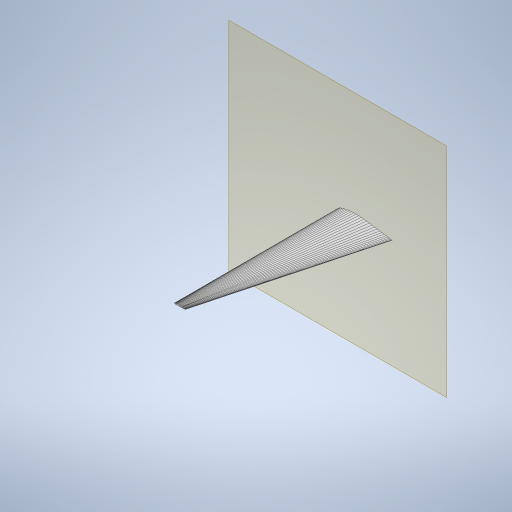
# Autodesk Inventor part: Część3
Saved by Autodesk Inventor 2023 (Build 270158000, 158)
## iProperties
Created: 2024-01-30
Part Number: Część3
Material: Ogólny
Document SubType Name: Modeling
Designer: domin
Density: 1 g/cm^3
Appearance: Domyślna
Author: domin
Autodesk Inventor part; units mm, degrees
ref_plane "YZ Plane" through (0, 0, 0) normal (1, 0, 0) x (0, 1, 0)
ref_plane "XZ Plane" through (0, 0, 0) normal (0, 1, 0) x (-1, 0, 0)
sketch "Szkic1" plane through (0, 0, 0) normal (0, 0, 1) x (1, 0, 0)
  line L0 (1, 0) -> (0.9965, 0.0005)
  line L1 (0.9965, 0.0005) -> (0.9863, 0.002)
  line L2 (0.9863, 0.002) -> (0.9701, 0.0049)
  line L3 (0.9701, 0.0049) -> (0.9487, 0.0088)
  line L4 (0.9487, 0.0088) -> (0.9224, 0.0134)
  line L5 (0.9224, 0.0134) -> (0.8913, 0.0184)
  line L6 (0.8913, 0.0184) -> (0.8558, 0.024)
  line L7 (0.8558, 0.024) -> (0.8163, 0.0301)
  line L8 (0.8163, 0.0301) -> (0.7736, 0.0367)
  line L9 (0.7736, 0.0367) -> (0.7281, 0.0435)
  line L10 (0.7281, 0.0435) -> (0.6804, 0.0506)
  line L11 (0.6804, 0.0506) -> (0.6313, 0.0576)
  line L12 (0.6313, 0.0576) -> (0.5814, 0.0644)
  line L13 (0.5814, 0.0644) -> (0.5313, 0.0708)
  line L14 (0.5313, 0.0708) -> (0.4817, 0.0764)
  line L15 (0.4817, 0.0764) -> (0.4331, 0.0808)
  line L16 (0.4331, 0.0808) -> (0.3857, 0.0836)
  line L17 (0.3857, 0.0836) -> (0.3398, 0.0848)
  line L18 (0.3398, 0.0848) -> (0.2957, 0.0843)
  line L19 (0.2957, 0.0843) -> (0.2536, 0.0821)
  line L20 (0.2536, 0.0821) -> (0.2137, 0.0782)
  line L21 (0.2137, 0.0782) -> (0.1762, 0.073)
  line L22 (0.1762, 0.073) -> (0.1416, 0.0667)
  line L23 (0.1416, 0.0667) -> (0.1102, 0.0594)
  line L24 (0.1102, 0.0594) -> (0.0823, 0.0514)
  line L25 (0.0823, 0.0514) -> (0.0581, 0.0428)
  line L26 (0.0581, 0.0428) -> (0.0379, 0.0338)
  line L27 (0.0379, 0.0338) -> (0.0219, 0.0247)
  line L28 (0.0219, 0.0247) -> (0.0102, 0.0157)
  line L29 (0.0102, 0.0157) -> (0.0028, 0.0071)
  line L30 (0.0028, 0.0071) -> (0, -0.0001)
  line L31 (0, -0.0001) -> (0.003, -0.0063)
  line L32 (0.003, -0.0063) -> (0.0121, -0.012)
  line L33 (0.0121, -0.012) -> (0.0263, -0.0175)
  line L34 (0.0263, -0.0175) -> (0.0454, -0.0223)
  line L35 (0.0454, -0.0223) -> (0.0694, -0.0265)
  line L36 (0.0694, -0.0265) -> (0.0981, -0.0299)
  line L37 (0.0981, -0.0299) -> (0.1311, -0.0326)
  line L38 (0.1311, -0.0326) -> (0.1682, -0.0345)
  line L39 (0.1682, -0.0345) -> (0.2089, -0.0357)
  line L40 (0.2089, -0.0357) -> (0.2529, -0.0361)
  line L41 (0.2529, -0.0361) -> (0.2997, -0.0359)
  line L42 (0.2997, -0.0359) -> (0.3486, -0.0349)
  line L43 (0.3486, -0.0349) -> (0.3994, -0.033)
  line L44 (0.3994, -0.033) -> (0.4517, -0.0304)
  line L45 (0.4517, -0.0304) -> (0.505, -0.0274)
  line L46 (0.505, -0.0274) -> (0.5586, -0.0243)
  line L47 (0.5586, -0.0243) -> (0.6119, -0.021)
  line L48 (0.6119, -0.021) -> (0.6641, -0.0179)
  line L49 (0.6641, -0.0179) -> (0.7147, -0.0149)
  line L50 (0.7147, -0.0149) -> (0.7628, -0.0121)
  line L51 (0.7628, -0.0121) -> (0.808, -0.0096)
  line L52 (0.808, -0.0096) -> (0.8495, -0.0074)
  line L53 (0.8495, -0.0074) -> (0.8868, -0.0056)
  line L54 (0.8868, -0.0056) -> (0.9194, -0.0039)
  line L55 (0.9194, -0.0039) -> (0.947, -0.0024)
  line L56 (0.947, -0.0024) -> (0.9693, -0.0011)
  line L57 (0.9693, -0.0011) -> (0.986, -0.0003)
  line L58 (0.986, -0.0003) -> (0.9964, 0)
  line L59 (0.9964, 0) -> (1, 0)
  point P0 (0, 0)
  dimension "d0" = 7.265
  dimension "d1" = 178.531
  dimension "d2" = 8.69
  dimension "d3" = 177.182
  dimension "d4" = 169.921
  dimension "d5" = 176.889
  dimension "d6" = 169.375
  dimension "d7" = 2.564
  dimension "d8" = 169.6
  dimension "d9" = 1.94
  dimension "d10" = 10.161
  dimension "d11" = 1.679
  dimension "d12" = 10.163
  dimension "d13" = 1.544
  dimension "d14" = 169.716
  dimension "d15" = 1.444
  dimension "d16" = 169.577
  dimension "d17" = 1.307
  dimension "d18" = 169.455
  dimension "d19" = 1.131
  dimension "d20" = 169.349
  dimension "d21" = 0.893
  dimension "d22" = 169.285
  dimension "d23" = 0.513
  dimension "d24" = 169.267
  dimension "d25" = 0.008
  dimension "d26" = 169.332
  dimension "d27" = 0.835
  dimension "d28" = 169.514
  dimension "d29" = 2.13
  dimension "d30" = 10.09
  dimension "d31" = 3.799
  dimension "d32" = 9.352
  dimension "d33" = 5.753
  dimension "d34" = 8.423
  dimension "d35" = 172.046
  dimension "d36" = 7.571
  dimension "d37" = 169.676
  dimension "d38" = 167.212
  dimension "d39" = 6.666
  dimension "d40" = 164.847
  dimension "d41" = 5.621
  dimension "d42" = 162.409
  dimension "d43" = 4.316
  dimension "d44" = 159.75
  dimension "d45" = 2.659
  dimension "d46" = 156.733
  dimension "d47" = 0.455
  dimension "d48" = 153.128
  dimension "d49" = 2.546
  dimension "d50" = 148.712
  dimension "d51" = 6.919
  dimension "d52" = 143.002
  dimension "d53" = 13.822
  dimension "d54" = 135.169
  dimension "d55" = 25.215
  dimension "d56" = 123.591
  dimension "d57" = 56.283
  dimension "d58" = 103.678
  dimension "d59" = 0.1265
  dimension "d60" = 0
  dimension "d61" = 0.1517
  dimension "d62" = 0.0248
  dimension "d63" = 0.1746
  constraints: 120 end point, 1 horizontal
  measures "d0" angle of L0 L59
  measures "d1" angle of L0 L1
  measures "d2" angle of L0 L58
  measures "d3" angle of L0 L2
  measures "d4" angle of L0 L57
  measures "d5" angle of L0 L3
  measures "d6" angle of L0 L56
  measures "d7" angle of L0 L4
  measures "d8" angle of L0 L55
  measures "d9" angle of L0 L5
  measures "d10" angle of L0 L54
  measures "d11" angle of L0 L6
  measures "d12" angle of L0 L53
  measures "d13" angle of L0 L7
  measures "d14" angle of L0 L52
  measures "d15" angle of L0 L8
  measures "d16" angle of L0 L51
  measures "d17" angle of L0 L9
  measures "d18" angle of L0 L50
  measures "d19" angle of L0 L10
  measures "d20" angle of L0 L49
  measures "d21" angle of L0 L11
  measures "d22" angle of L0 L48
  measures "d23" angle of L0 L12
  measures "d24" angle of L0 L47
  measures "d25" angle of L0 L13
  measures "d26" angle of L0 L46
  measures "d27" angle of L0 L14
  measures "d28" angle of L0 L45
  measures "d29" angle of L0 L15
  measures "d30" angle of L0 L44
  measures "d31" angle of L0 L16
  measures "d32" angle of L0 L43
  measures "d33" angle of L0 L17
  measures "d34" angle of L0 L42
  measures "d35" angle of L0 L18
  measures "d36" angle of L0 L41
  measures "d37" angle of L0 L19
  measures "d38" angle of L0 L20
  measures "d39" angle of L0 L40
  measures "d40" angle of L0 L21
  measures "d41" angle of L0 L39
  measures "d42" angle of L0 L22
  measures "d43" angle of L0 L38
  measures "d44" angle of L0 L23
  measures "d45" angle of L0 L37
  measures "d46" angle of L0 L24
  measures "d47" angle of L0 L36
  measures "d48" angle of L0 L25
  measures "d49" angle of L0 L35
  measures "d50" angle of L0 L26
  measures "d51" angle of L0 L34
  measures "d52" angle of L0 L27
  measures "d53" angle of L0 L33
  measures "d54" angle of L0 L28
  measures "d55" angle of L0 L32
  measures "d56" angle of L0 L29
  measures "d57" angle of L0 L31
  measures "d58" angle of L0 L30
  measures "d59" distance from line of point (0, 0) L0
  measures "d60" distance from line of point (0, 0) L59
  measures "d61" distance from line of point (0, 0) L1
  measures "d62" distance from line of point (0, 0) L58
  measures "d63" distance from line of point (0, 0) L2
ref_plane "Płaszczyzna konstrukcyjna1" through (0, 0, -15) normal (0, 0, 1) x (1, 0, 0)
sketch "Szkic2" plane through (0, 0, -15) normal (0, 0, 1) x (1, 0, 0)
  line L0 (5, 0) -> (4.9824, 0.0023)
  line L1 (4.9824, 0.0023) -> (4.9313, 0.0101)
  line L2 (4.9313, 0.0101) -> (4.8506, 0.0244)
  line L3 (4.8506, 0.0244) -> (4.7435, 0.044)
  line L4 (4.7435, 0.044) -> (4.6119, 0.0668)
  line L5 (4.6119, 0.0668) -> (4.4564, 0.092)
  line L6 (4.4564, 0.092) -> (4.2788, 0.12)
  line L7 (4.2788, 0.12) -> (4.0817, 0.1506)
  line L8 (4.0817, 0.1506) -> (3.8679, 0.1833)
  line L9 (3.8679, 0.1833) -> (3.6403, 0.2176)
  line L10 (3.6403, 0.2176) -> (3.4022, 0.2528)
  line L11 (3.4022, 0.2528) -> (3.1566, 0.288)
  line L12 (3.1566, 0.288) -> (2.9069, 0.322)
  line L13 (2.9069, 0.322) -> (2.6565, 0.354)
  line L14 (2.6565, 0.354) -> (2.4085, 0.3819)
  line L15 (2.4085, 0.3819) -> (2.1653, 0.4037)
  line L16 (2.1653, 0.4037) -> (1.9284, 0.4181)
  line L17 (1.9284, 0.4181) -> (1.6991, 0.4242)
  line L18 (1.6991, 0.4242) -> (1.4787, 0.4215)
  line L19 (1.4787, 0.4215) -> (1.2682, 0.4103)
  line L20 (1.2682, 0.4103) -> (1.0686, 0.3909)
  line L21 (1.0686, 0.3909) -> (0.8812, 0.365)
  line L22 (0.8812, 0.365) -> (0.7081, 0.3335)
  line L23 (0.7081, 0.3335) -> (0.5509, 0.2972)
  line L24 (0.5509, 0.2972) -> (0.4113, 0.2571)
  line L25 (0.4113, 0.2571) -> (0.2904, 0.2141)
  line L26 (0.2904, 0.2141) -> (0.1895, 0.1691)
  line L27 (0.1895, 0.1691) -> (0.1094, 0.1234)
  line L28 (0.1094, 0.1234) -> (0.0508, 0.0783)
  line L29 (0.0508, 0.0783) -> (0.014, 0.0357)
  line L30 (0.014, 0.0357) -> (0, -0.0007)
  line L31 (0, -0.0007) -> (0.0152, -0.0313)
  line L32 (0.0152, -0.0313) -> (0.0606, -0.0602)
  line L33 (0.0606, -0.0602) -> (0.1314, -0.0875)
  line L34 (0.1314, -0.0875) -> (0.2271, -0.1117)
  line L35 (0.2271, -0.1117) -> (0.3472, -0.1325)
  line L36 (0.3472, -0.1325) -> (0.4904, -0.1496)
  line L37 (0.4904, -0.1496) -> (0.6555, -0.1628)
  line L38 (0.6555, -0.1628) -> (0.8408, -0.1724)
  line L39 (0.8408, -0.1724) -> (1.0447, -0.1783)
  line L40 (1.0447, -0.1783) -> (1.2646, -0.1806)
  line L41 (1.2646, -0.1806) -> (1.4983, -0.1793)
  line L42 (1.4983, -0.1793) -> (1.743, -0.1744)
  line L43 (1.743, -0.1744) -> (1.9969, -0.1651)
  line L44 (1.9969, -0.1651) -> (2.2583, -0.1522)
  line L45 (2.2583, -0.1522) -> (2.5248, -0.1372)
  line L46 (2.5248, -0.1372) -> (2.793, -0.1212)
  line L47 (2.793, -0.1212) -> (3.0595, -0.1051)
  line L48 (3.0595, -0.1051) -> (3.3207, -0.0893)
  line L49 (3.3207, -0.0893) -> (3.5734, -0.0744)
  line L50 (3.5734, -0.0744) -> (3.8142, -0.0606)
  line L51 (3.8142, -0.0606) -> (4.0398, -0.0481)
  line L52 (4.0398, -0.0481) -> (4.2474, -0.0372)
  line L53 (4.2474, -0.0372) -> (4.4341, -0.0278)
  line L54 (4.4341, -0.0278) -> (4.5971, -0.0195)
  line L55 (4.5971, -0.0195) -> (4.7349, -0.012)
  line L56 (4.7349, -0.012) -> (4.8465, -0.0054)
  line L57 (4.8465, -0.0054) -> (4.9299, -0.0013)
  line L58 (4.9299, -0.0013) -> (4.9822, 0)
  line L59 (4.9822, 0) -> (5, 0)
  point P0 (0, 0)
  point P1 (0, 0.0003)
  dimension "d122" = 7.265
  dimension "d123" = 178.531
  dimension "d124" = 8.69
  dimension "d125" = 177.182
  dimension "d126" = 169.921
  dimension "d127" = 176.889
  dimension "d128" = 169.375
  dimension "d129" = 2.564
  dimension "d130" = 169.6
  dimension "d131" = 1.94
  dimension "d132" = 10.161
  dimension "d133" = 1.679
  dimension "d134" = 10.163
  dimension "d135" = 1.544
  dimension "d136" = 169.716
  dimension "d137" = 1.444
  dimension "d138" = 169.577
  dimension "d139" = 1.307
  dimension "d140" = 169.455
  dimension "d141" = 1.131
  dimension "d142" = 169.349
  dimension "d143" = 0.893
  dimension "d144" = 169.285
  dimension "d145" = 0.513
  dimension "d146" = 169.267
  dimension "d147" = 0.008
  dimension "d148" = 169.332
  dimension "d149" = 0.835
  dimension "d150" = 169.514
  dimension "d151" = 2.13
  dimension "d152" = 10.09
  dimension "d153" = 3.799
  dimension "d154" = 9.352
  dimension "d155" = 5.753
  dimension "d156" = 8.423
  dimension "d157" = 172.046
  dimension "d158" = 7.571
  dimension "d159" = 169.676
  dimension "d160" = 167.212
  dimension "d161" = 6.666
  dimension "d162" = 164.847
  dimension "d163" = 5.621
  dimension "d164" = 162.409
  dimension "d165" = 4.316
  dimension "d166" = 159.75
  dimension "d167" = 2.659
  dimension "d168" = 156.733
  dimension "d169" = 0.455
  dimension "d170" = 153.128
  dimension "d171" = 2.546
  dimension "d172" = 148.712
  dimension "d173" = 6.919
  dimension "d174" = 143.002
  dimension "d175" = 13.822
  dimension "d176" = 135.169
  dimension "d177" = 25.215
  dimension "d178" = 123.591
  dimension "d179" = 56.283
  dimension "d180" = 103.678
  dimension "d181" = 0.632
  dimension "d182" = -0.0003
  dimension "d183" = 0.7585
  dimension "d184" = 0.1242
  dimension "d185" = 0.873
  constraints: 120 end point, 1 horizontal
  measures "d122" angle of L0 L59
  measures "d123" angle of L0 L1
  measures "d124" angle of L0 L58
  measures "d125" angle of L0 L2
  measures "d126" angle of L0 L57
  measures "d127" angle of L0 L3
  measures "d128" angle of L0 L56
  measures "d129" angle of L0 L4
  measures "d130" angle of L0 L55
  measures "d131" angle of L0 L5
  measures "d132" angle of L0 L54
  measures "d133" angle of L0 L6
  measures "d134" angle of L0 L53
  measures "d135" angle of L0 L7
  measures "d136" angle of L0 L52
  measures "d137" angle of L0 L8
  measures "d138" angle of L0 L51
  measures "d139" angle of L0 L9
  measures "d140" angle of L0 L50
  measures "d141" angle of L0 L10
  measures "d142" angle of L0 L49
  measures "d143" angle of L0 L11
  measures "d144" angle of L0 L48
  measures "d145" angle of L0 L12
  measures "d146" angle of L0 L47
  measures "d147" angle of L0 L13
  measures "d148" angle of L0 L46
  measures "d149" angle of L0 L14
  measures "d150" angle of L0 L45
  measures "d151" angle of L0 L15
  measures "d152" angle of L0 L44
  measures "d153" angle of L0 L16
  measures "d154" angle of L0 L43
  measures "d155" angle of L0 L17
  measures "d156" angle of L0 L42
  measures "d157" angle of L0 L18
  measures "d158" angle of L0 L41
  measures "d159" angle of L0 L19
  measures "d160" angle of L0 L20
  measures "d161" angle of L0 L40
  measures "d162" angle of L0 L21
  measures "d163" angle of L0 L39
  measures "d164" angle of L0 L22
  measures "d165" angle of L0 L38
  measures "d166" angle of L0 L23
  measures "d167" angle of L0 L37
  measures "d168" angle of L0 L24
  measures "d169" angle of L0 L36
  measures "d170" angle of L0 L25
  measures "d171" angle of L0 L35
  measures "d172" angle of L0 L26
  measures "d173" angle of L0 L34
  measures "d174" angle of L0 L27
  measures "d175" angle of L0 L33
  measures "d176" angle of L0 L28
  measures "d177" angle of L0 L32
  measures "d178" angle of L0 L29
  measures "d179" angle of L0 L31
  measures "d180" angle of L0 L30
  measures "d181" distance from line of point (0, 0) L0
  measures "d182" distance from line of point (0, 0) L59
  measures "d183" distance from line of point (0, 0) L1
  measures "d184" distance from line of point (0, 0) L58
  measures "d185" distance from line of point (0, 0) L2
loft "Wyciągnięcie złożone1" add profiles "Szkic1", "Szkic2"
